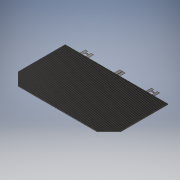
# Autodesk Inventor part: Part1
Saved by Autodesk Inventor 2017 (Build 210142000, 142)
## iProperties
Created: 2018-02-04
Part Number: Part1
Material: Glass
Document SubType Name: Modeling
Designer: Bradley
Density: 2.18 g/cm^3
Appearance: Semi-Polished
Author: Bradley
Autodesk Inventor part; units mm, degrees
ref_plane "YZ Plane" through (0, 0, 0) normal (1, 0, 0) x (0, 1, 0)
ref_plane "XZ Plane" through (0, 0, 0) normal (0, 1, 0) x (-1, 0, 0)
ref_plane "XY Plane" through (0, 0, 0) normal (0, 0, 1) x (1, 0, 0)
sketch "Sketch1" plane through (0, 0, 0) normal (0, 0, 1) x (1, 0, 0)
  line L0 (-26.5, -19.825) -> (26.5, -19.825)
  line L1 (34.5, -11.825) -> (34.5, 19.825)
  line L2 (34.5, 19.825) -> (-34.5, 19.825)
  line L3 (-34.5, 19.825) -> (-34.5, -11.825)
  line L4 (-34.5, -19.825) -> (34.5, 19.825) construction
  line L5 (34.5, -19.825) -> (-34.5, 19.825) construction
  line L6 (-34.5, -11.825) -> (-26.5, -19.825)
  line L7 (34.5, -11.825) -> (26.5, -19.825)
  point P0 (0, 0)
  dimension "d0" = 69
  dimension "d1" = 39.65
  dimension "d2" = 8
  dimension "d3" = 8
  dimension "d4" = 8
  dimension "d5" = 8
  constraints: 16 end point, 4 point on line, 2 midpoint, 2 parallel, 1 horizontal, 1 perpendicular
  measures "d0" distance of L2.end L1.end
  measures "d1" distance of L2.end L4.start
  measures "d2" distance of L3.end L4.start
  measures "d3" distance of L0.start L4.start
  measures "d4" distance of L1.start L5.start
  measures "d5" distance of L0.end L5.start
extrude "Extrusion1" add sketch "Sketch1" along normal mid plane 0.4
sketch "Sketch2" plane through (0, 0, -0.2) normal (0, 0, -1) x (-1, 0, 0)
  line L0 (-34.5, 19.825) -> (-34.5, -11.825) projected
  line L1 (-34.5, -11.825) -> (-26.5, -19.825) projected
  line L2 (-26.5, -19.825) -> (26.5, -19.825) projected
  line L3 (26.5, -19.825) -> (34.5, -11.825) projected
  line L4 (34.5, -11.825) -> (34.5, 19.825) projected
  line L5 (34.5, 19.825) -> (-34.5, 19.825) projected
  line L6 (-34.5, 19.825) -> (34.5, 19.825) projected
  line L7 (-3.125, 19.825) -> (3.125, 19.825)
  line L8 (3.125, 19.825) -> (3.125, 13.575)
  line L9 (3.125, 13.575) -> (-3.125, 13.575)
  line L10 (-3.125, 13.575) -> (-3.125, 19.825)
  point P0 (0, 0)
  point P1 (0, 13.575)
  dimension "d8" = 6.25
  constraints: 8 end point, 2 parallel, 2 perpendicular, 1 horizontal, 1 midpoint, 1 point on line, 1 vertical alignment
  measures "d8" distance of L8.end L9.end
extrude "Extrusion2" add sketch "Sketch2" along normal blind 0.1 contours L5 L8 L9 L10
sketch "Sketch3" plane through (-34.5, 19.825, 0.2) normal (0, 1, 0) x (1, 0, 0)
  line L0 (0, 0) -> (0, 0.4) projected
  line L1 (69, 0) -> (0, 0) projected
  line L2 (69, 0.4) -> (69, 0) projected
  line L3 (37.625, 0.4) -> (69, 0.4) projected
  line L4 (37.625, 0.4) -> (37.625, 0.5) projected
  line L5 (31.375, 0.5) -> (37.625, 0.5) projected
  line L6 (31.375, 0.4) -> (31.375, 0.5) projected
  line L7 (0, 0.4) -> (31.375, 0.4) projected
  line L8 (53.875, 0.32) -> (59.475, 0.32)
  line L9 (59.475, 0.32) -> (59.475, 0.38)
  line L10 (59.475, 0.38) -> (53.875, 0.38)
  line L11 (53.875, 0.38) -> (53.875, 0.32)
  line L12 (9.525, 0.32) -> (15.125, 0.32)
  line L13 (15.125, 0.32) -> (15.125, 0.38)
  line L14 (15.125, 0.38) -> (9.525, 0.38)
  line L15 (9.525, 0.38) -> (9.525, 0.32)
  line L16 (8, 0) -> (61, 0) construction
  line L17 (34.5, 0) -> (34.5, 0.5) construction
  line L18 (32.625, 0.32) -> (36.375, 0.32)
  line L19 (36.375, 0.32) -> (36.375, 0.38)
  line L20 (36.375, 0.38) -> (32.625, 0.38)
  line L21 (32.625, 0.38) -> (32.625, 0.32)
  point P0 (34.5, 0.2)
  point P1 (34.5, 0.32)
  dimension "d11" = 5.6
  dimension "d12" = 0.06
  dimension "d13" = 38.75
  dimension "d14" = 0.02
  dimension "d15" = 3.75
  constraints: 26 end point, 6 parallel, 4 collinear, 3 horizontal, 3 midpoint, 3 perpendicular, 1 vertical alignment, 2 other
  measures "d11" distance of L10.end L9.end
  measures "d12" distance of L10.end L8.start
  measures "d13" distance between parallel lines of L13 L11
  measures "d14" distance between parallel lines of L3 L10
  measures "d15" distance of L19.end L20.end
extrude "Extrusion3" add sketch "Sketch3" along normal blind 10.5 contours L11 L10 L9 L8 | L15 L14 L13 L12 | L21 L20 L19 L18
sketch "Sketch4" plane through (-24.975, 19.825, -0.12) normal (0, 0, 1) x (1, 0, 0)
  line L0 (5.6, 0) -> (0, 0) projected
  line L1 (5.6, 0) -> (5.6, 10.5) projected
  line L2 (0, 10.5) -> (5.6, 10.5) projected
  line L3 (0, 0) -> (0, 10.5) projected
  line L4 (-9.525, 0) -> (21.85, 0) projected
  line L5 (1.6, 0) -> (4, 0)
  line L6 (4, 0) -> (4, 1.9)
  line L7 (4, 1.9) -> (1.6, 1.9)
  line L8 (1.6, 1.9) -> (1.6, 0)
  line L9 (1.6, 2.65) -> (4, 2.65)
  line L10 (4, 2.65) -> (4, 5.9)
  line L11 (4, 5.9) -> (1.6, 5.9)
  line L12 (1.6, 5.9) -> (1.6, 2.65)
  line L13 (0, 10.5) -> (5.6, 10.5) projected
  line L14 (1.6, 10.5) -> (4, 10.5)
  line L15 (4, 10.5) -> (4, 6.65)
  line L16 (4, 6.65) -> (1.6, 6.65)
  line L17 (1.6, 6.65) -> (1.6, 10.5)
  point P0 (24.975, -19.825)
  point P1 (2.8, 10.5)
  dimension "d18" = 1.6
  dimension "d19" = 0.75
  dimension "d20" = 0.75
  dimension "d21" = 3.25
  dimension "d22" = 1.9
  constraints: 24 end point, 6 parallel, 6 point on line, 3 horizontal, 3 perpendicular, 2 midpoint
  measures "d18" distance between parallel lines of L3 L17
  measures "d19" distance between parallel lines of L11 L16
  measures "d20" distance between parallel lines of L7 L9
  measures "d21" distance of L9.end L10.end
  measures "d22" distance of L5.end L6.end
extrude "Extrusion4" cut sketch "Sketch4" against normal through all contours L0 L8 L7 L6 | L15 L16 L17 L2 | L12 L11 L10 L9
sketch "Sketch5" plane through (-1.875, 19.825, -0.12) normal (0, 0, 1) x (1, 0, 0)
  line L0 (3.75, 0) -> (0, 0) projected
  line L1 (3.75, 0) -> (3.75, 10.5) projected
  line L2 (0, 10.5) -> (3.75, 10.5) projected
  line L3 (0, 0) -> (0, 10.5) projected
  line L4 (0, 10.5) -> (3.75, 10.5) projected
  line L5 (1.75, 10.5) -> (2, 10.5)
  line L6 (2, 10.5) -> (2, 7.25)
  line L7 (2, 7.25) -> (1.75, 7.25)
  line L8 (1.75, 7.25) -> (1.75, 10.5)
  line L9 (0, 0) -> (3.75, 0) projected
  line L10 (1.75, 0) -> (2, 0)
  line L11 (2, 0) -> (2, 6.25)
  line L12 (2, 6.25) -> (1.75, 6.25)
  line L13 (1.75, 6.25) -> (1.75, 0)
  point P0 (1.875, -19.825)
  point P1 (1.875, 10.5)
  point P2 (1.875, 10.5)
  dimension "d25" = 1.75
  dimension "d26" = 1
  dimension "d27" = 6.25
  constraints: 16 end point, 4 midpoint, 4 parallel, 4 point on line, 2 horizontal, 2 perpendicular
  measures "d25" distance between parallel lines of L3 L8
  measures "d26" distance between parallel lines of L12 L7
  measures "d27" distance of L10.end L11.end
extrude "Extrusion5" cut sketch "Sketch5" against normal through all contours L0 L13 L12 L11 | L6 L7 L8 L2
mirror "Mirror1" about plane through (0, 0, 0) normal (1, 0, 0) of "Extrusion4"
sketch "Sketch6" plane through (0, 0, 0.2) normal (0, 0, 1) x (1, 0, 0)
  line L0 (34.5, -11.825) -> (34.5, 19.825) projected
  line L1 (34.5, 19.825) -> (-34.5, 19.825) projected
  line L2 (-34.5, 19.825) -> (-34.5, -11.825) projected
  line L3 (-34.5, -11.825) -> (-26.5, -19.825) projected
  line L4 (-26.5, -19.825) -> (26.5, -19.825) projected
  line L5 (26.5, -19.825) -> (34.5, -11.825) projected
  line L6 (33.9, 19.325) -> (34.1, 19.325)
  line L7 (34.1, 19.325) -> (34.1, -19.625)
  line L8 (34.1, -19.625) -> (33.9, -19.625)
  line L9 (33.9, -19.625) -> (33.9, 19.325)
  point P0 (0, 0)
  dimension "d30" = 0.2
  dimension "d31" = 0.5
  dimension "d32" = 0.2
  dimension "d33" = 33.9
  constraints: 8 end point, 2 parallel, 1 horizontal, 1 perpendicular
  measures "d30" distance between parallel lines of L8 L4
  measures "d31" distance between parallel lines of L1 L6
  measures "d32" distance of L6.start L6.end
  measures "d33" distance from line of point (0, 0) L9
extrude "Extrusion6" add sketch "Sketch6" along normal blind 0.01 contours L7 L8 L9 L5 | L5 L9 L6 L7
pattern_linear "Rectangular Pattern1" count 69 spacing 1 along (-1, 0, 0) of "Extrusion6"
sketch "Sketch7" plane through (0, 0, 0.2) normal (0, 0, 1) x (1, 0, 0)
  line L0 (-33.9, 19.325) -> (-33.9, -12.425) projected
  line L1 (-33.9, -12.425) -> (-33.1, -13.225) projected
  line L2 (-33.1, -13.225) -> (-33.1, 19.325) projected
  line L3 (-33.1, 19.325) -> (-32.9, 19.325) projected
  line L4 (-32.9, 19.325) -> (-32.9, -13.425) projected
  line L5 (-32.9, -13.425) -> (-32.1, -14.225) projected
  line L6 (-32.1, -14.225) -> (-32.1, 19.325) projected
  line L7 (-32.1, 19.325) -> (-31.9, 19.325) projected
  line L8 (-31.9, 19.325) -> (-31.9, -14.425) projected
  line L9 (-31.9, -14.425) -> (-31.1, -15.225) projected
  line L10 (-31.1, -15.225) -> (-31.1, 19.325) projected
  line L11 (-31.1, 19.325) -> (-30.9, 19.325) projected
  line L12 (-30.9, 19.325) -> (-30.9, -15.425) projected
  line L13 (-30.9, -15.425) -> (-30.1, -16.225) projected
  line L14 (-30.1, -16.225) -> (-30.1, 19.325) projected
  line L15 (-30.1, 19.325) -> (-29.9, 19.325) projected
  line L16 (-29.9, 19.325) -> (-29.9, -16.425) projected
  line L17 (-29.9, -16.425) -> (-29.1, -17.225) projected
  line L18 (-29.1, -17.225) -> (-29.1, 19.325) projected
  line L19 (-29.1, 19.325) -> (-28.9, 19.325) projected
  line L20 (-28.9, 19.325) -> (-28.9, -17.425) projected
  line L21 (-28.9, -17.425) -> (-28.1, -18.225) projected
  line L22 (-28.1, -18.225) -> (-28.1, 19.325) projected
  line L23 (-28.1, 19.325) -> (-27.9, 19.325) projected
  line L24 (-27.9, 19.325) -> (-27.9, -18.425) projected
  line L25 (-27.9, -18.425) -> (-27.1, -19.225) projected
  line L26 (-27.1, -19.225) -> (-27.1, 19.325) projected
  line L27 (-27.1, 19.325) -> (-26.9, 19.325) projected
  line L28 (-26.9, 19.325) -> (-26.9, -19.425) projected
  line L29 (-26.9, -19.425) -> (-26.5, -19.825) projected
  line L30 (-26.5, -19.825) -> (26.5, -19.825) projected
  line L31 (26.5, -19.825) -> (26.9, -19.425) projected
  line L32 (26.9, -19.425) -> (26.9, 19.325) projected
  line L33 (26.9, 19.325) -> (27.1, 19.325) projected
  line L34 (27.1, 19.325) -> (27.1, -19.225) projected
  line L35 (27.1, -19.225) -> (27.9, -18.425) projected
  line L36 (27.9, -18.425) -> (27.9, 19.325) projected
  line L37 (27.9, 19.325) -> (28.1, 19.325) projected
  line L38 (28.1, 19.325) -> (28.1, -18.225) projected
  line L39 (28.1, -18.225) -> (28.9, -17.425) projected
  line L40 (28.9, -17.425) -> (28.9, 19.325) projected
  line L41 (28.9, 19.325) -> (29.1, 19.325) projected
  line L42 (29.1, 19.325) -> (29.1, -17.225) projected
  line L43 (29.1, -17.225) -> (29.9, -16.425) projected
  line L44 (29.9, -16.425) -> (29.9, 19.325) projected
  line L45 (29.9, 19.325) -> (30.1, 19.325) projected
  line L46 (30.1, 19.325) -> (30.1, -16.225) projected
  line L47 (30.1, -16.225) -> (30.9, -15.425) projected
  line L48 (30.9, -15.425) -> (30.9, 19.325) projected
  line L49 (30.9, 19.325) -> (31.1, 19.325) projected
  line L50 (31.1, 19.325) -> (31.1, -15.225) projected
  line L51 (31.1, -15.225) -> (31.9, -14.425) projected
  line L52 (31.9, -14.425) -> (31.9, 19.325) projected
  line L53 (31.9, 19.325) -> (32.1, 19.325) projected
  line L54 (32.1, 19.325) -> (32.1, -14.225) projected
  line L55 (32.1, -14.225) -> (32.9, -13.425) projected
  line L56 (32.9, -13.425) -> (32.9, 19.325) projected
  line L57 (32.9, 19.325) -> (33.1, 19.325) projected
  line L58 (33.1, 19.325) -> (33.1, -13.225) projected
  line L59 (33.1, -13.225) -> (33.9, -12.425) projected
  line L60 (33.9, -12.425) -> (33.9, 19.325) projected
  line L61 (33.9, 19.325) -> (34.1, 19.325) projected
  line L62 (34.1, 19.325) -> (34.1, -12.225) projected
  line L63 (34.1, -12.225) -> (34.5, -11.825) projected
  line L64 (34.5, -11.825) -> (34.5, 19.825) projected
  line L65 (34.5, 19.825) -> (-34.5, 19.825) projected
  line L66 (-34.5, 19.825) -> (-34.5, -11.825) projected
  line L67 (-34.5, -11.825) -> (-34.1, -12.225) projected
  line L68 (-34.1, -12.225) -> (-34.1, 19.325) projected
  line L69 (-34.1, 19.325) -> (-33.9, 19.325) projected
  line L70 (-25.9, 19.325) -> (-25.9, -19.625) projected
  line L71 (-25.9, -19.625) -> (-26.1, -19.625) projected
  line L72 (-26.1, -19.625) -> (-26.1, 19.325) projected
  line L73 (-26.1, 19.325) -> (-25.9, 19.325) projected
  line L74 (-24.9, 19.325) -> (-24.9, -19.625) projected
  line L75 (-24.9, -19.625) -> (-25.1, -19.625) projected
  line L76 (-25.1, -19.625) -> (-25.1, 19.325) projected
  line L77 (-25.1, 19.325) -> (-24.9, 19.325) projected
  line L78 (-23.9, 19.325) -> (-23.9, -19.625) projected
  line L79 (-23.9, -19.625) -> (-24.1, -19.625) projected
  line L80 (-24.1, -19.625) -> (-24.1, 19.325) projected
  line L81 (-24.1, 19.325) -> (-23.9, 19.325) projected
  line L82 (-22.9, 19.325) -> (-22.9, -19.625) projected
  line L83 (-22.9, -19.625) -> (-23.1, -19.625) projected
  line L84 (-23.1, -19.625) -> (-23.1, 19.325) projected
  line L85 (-23.1, 19.325) -> (-22.9, 19.325) projected
  line L86 (-21.9, 19.325) -> (-21.9, -19.625) projected
  line L87 (-21.9, -19.625) -> (-22.1, -19.625) projected
  line L88 (-22.1, -19.625) -> (-22.1, 19.325) projected
  line L89 (-22.1, 19.325) -> (-21.9, 19.325) projected
  line L90 (-20.9, 19.325) -> (-20.9, -19.625) projected
  line L91 (-20.9, -19.625) -> (-21.1, -19.625) projected
  line L92 (-21.1, -19.625) -> (-21.1, 19.325) projected
  line L93 (-21.1, 19.325) -> (-20.9, 19.325) projected
  line L94 (-19.9, 19.325) -> (-19.9, -19.625) projected
  line L95 (-19.9, -19.625) -> (-20.1, -19.625) projected
  line L96 (-20.1, -19.625) -> (-20.1, 19.325) projected
  line L97 (-20.1, 19.325) -> (-19.9, 19.325) projected
  line L98 (-18.9, 19.325) -> (-18.9, -19.625) projected
  line L99 (-18.9, -19.625) -> (-19.1, -19.625) projected
  line L100 (-19.1, -19.625) -> (-19.1, 19.325) projected
  line L101 (-19.1, 19.325) -> (-18.9, 19.325) projected
  line L102 (-17.9, 19.325) -> (-17.9, -19.625) projected
  line L103 (-17.9, -19.625) -> (-18.1, -19.625) projected
  line L104 (-18.1, -19.625) -> (-18.1, 19.325) projected
  line L105 (-18.1, 19.325) -> (-17.9, 19.325) projected
  line L106 (-16.9, 19.325) -> (-16.9, -19.625) projected
  line L107 (-16.9, -19.625) -> (-17.1, -19.625) projected
  line L108 (-17.1, -19.625) -> (-17.1, 19.325) projected
  line L109 (-17.1, 19.325) -> (-16.9, 19.325) projected
  line L110 (-15.9, 19.325) -> (-15.9, -19.625) projected
  line L111 (-15.9, -19.625) -> (-16.1, -19.625) projected
  line L112 (-16.1, -19.625) -> (-16.1, 19.325) projected
  line L113 (-16.1, 19.325) -> (-15.9, 19.325) projected
  line L114 (-14.9, 19.325) -> (-14.9, -19.625) projected
  line L115 (-14.9, -19.625) -> (-15.1, -19.625) projected
  line L116 (-15.1, -19.625) -> (-15.1, 19.325) projected
  line L117 (-15.1, 19.325) -> (-14.9, 19.325) projected
  line L118 (-13.9, 19.325) -> (-13.9, -19.625) projected
  line L119 (-13.9, -19.625) -> (-14.1, -19.625) projected
  line L120 (-14.1, -19.625) -> (-14.1, 19.325) projected
  line L121 (-14.1, 19.325) -> (-13.9, 19.325) projected
  line L122 (-12.9, 19.325) -> (-12.9, -19.625) projected
  line L123 (-12.9, -19.625) -> (-13.1, -19.625) projected
  line L124 (-13.1, -19.625) -> (-13.1, 19.325) projected
  line L125 (-13.1, 19.325) -> (-12.9, 19.325) projected
  line L126 (-11.9, 19.325) -> (-11.9, -19.625) projected
  line L127 (-11.9, -19.625) -> (-12.1, -19.625) projected
  line L128 (-12.1, -19.625) -> (-12.1, 19.325) projected
  line L129 (-12.1, 19.325) -> (-11.9, 19.325) projected
  line L130 (-10.9, 19.325) -> (-10.9, -19.625) projected
  line L131 (-10.9, -19.625) -> (-11.1, -19.625) projected
  line L132 (-11.1, -19.625) -> (-11.1, 19.325) projected
  line L133 (-11.1, 19.325) -> (-10.9, 19.325) projected
  line L134 (-9.9, 19.325) -> (-9.9, -19.625) projected
  line L135 (-9.9, -19.625) -> (-10.1, -19.625) projected
  line L136 (-10.1, -19.625) -> (-10.1, 19.325) projected
  line L137 (-10.1, 19.325) -> (-9.9, 19.325) projected
  line L138 (-8.9, 19.325) -> (-8.9, -19.625) projected
  line L139 (-8.9, -19.625) -> (-9.1, -19.625) projected
  line L140 (-9.1, -19.625) -> (-9.1, 19.325) projected
  line L141 (-9.1, 19.325) -> (-8.9, 19.325) projected
  line L142 (-7.9, 19.325) -> (-7.9, -19.625) projected
  line L143 (-7.9, -19.625) -> (-8.1, -19.625) projected
  line L144 (-8.1, -19.625) -> (-8.1, 19.325) projected
  line L145 (-8.1, 19.325) -> (-7.9, 19.325) projected
  line L146 (-6.9, 19.325) -> (-6.9, -19.625) projected
  line L147 (-6.9, -19.625) -> (-7.1, -19.625) projected
  line L148 (-7.1, -19.625) -> (-7.1, 19.325) projected
  line L149 (-7.1, 19.325) -> (-6.9, 19.325) projected
  line L150 (-5.9, 19.325) -> (-5.9, -19.625) projected
  line L151 (-5.9, -19.625) -> (-6.1, -19.625) projected
  line L152 (-6.1, -19.625) -> (-6.1, 19.325) projected
  line L153 (-6.1, 19.325) -> (-5.9, 19.325) projected
  line L154 (-4.9, 19.325) -> (-4.9, -19.625) projected
  line L155 (-4.9, -19.625) -> (-5.1, -19.625) projected
  line L156 (-5.1, -19.625) -> (-5.1, 19.325) projected
  line L157 (-5.1, 19.325) -> (-4.9, 19.325) projected
  line L158 (-3.9, 19.325) -> (-3.9, -19.625) projected
  line L159 (-3.9, -19.625) -> (-4.1, -19.625) projected
  line L160 (-4.1, -19.625) -> (-4.1, 19.325) projected
  line L161 (-4.1, 19.325) -> (-3.9, 19.325) projected
  line L162 (-2.9, 19.325) -> (-2.9, -19.625) projected
  line L163 (-2.9, -19.625) -> (-3.1, -19.625) projected
  line L164 (-3.1, -19.625) -> (-3.1, 19.325) projected
  line L165 (-3.1, 19.325) -> (-2.9, 19.325) projected
  line L166 (-1.9, 19.325) -> (-1.9, -19.625) projected
  line L167 (-1.9, -19.625) -> (-2.1, -19.625) projected
  line L168 (-2.1, -19.625) -> (-2.1, 19.325) projected
  line L169 (-2.1, 19.325) -> (-1.9, 19.325) projected
  line L170 (-0.9, 19.325) -> (-0.9, -19.625) projected
  line L171 (-0.9, -19.625) -> (-1.1, -19.625) projected
  line L172 (-1.1, -19.625) -> (-1.1, 19.325) projected
  line L173 (-1.1, 19.325) -> (-0.9, 19.325) projected
  line L174 (0.1, 19.325) -> (0.1, -19.625) projected
  line L175 (0.1, -19.625) -> (-0.1, -19.625) projected
  line L176 (-0.1, -19.625) -> (-0.1, 19.325) projected
  line L177 (-0.1, 19.325) -> (0.1, 19.325) projected
  line L178 (1.1, 19.325) -> (1.1, -19.625) projected
  line L179 (1.1, -19.625) -> (0.9, -19.625) projected
  line L180 (0.9, -19.625) -> (0.9, 19.325) projected
  line L181 (0.9, 19.325) -> (1.1, 19.325) projected
  line L182 (2.1, 19.325) -> (2.1, -19.625) projected
  line L183 (2.1, -19.625) -> (1.9, -19.625) projected
  line L184 (1.9, -19.625) -> (1.9, 19.325) projected
  line L185 (1.9, 19.325) -> (2.1, 19.325) projected
  line L186 (3.1, 19.325) -> (3.1, -19.625) projected
  line L187 (3.1, -19.625) -> (2.9, -19.625) projected
  line L188 (2.9, -19.625) -> (2.9, 19.325) projected
  line L189 (2.9, 19.325) -> (3.1, 19.325) projected
  line L190 (4.1, 19.325) -> (4.1, -19.625) projected
  line L191 (4.1, -19.625) -> (3.9, -19.625) projected
  line L192 (3.9, -19.625) -> (3.9, 19.325) projected
  line L193 (3.9, 19.325) -> (4.1, 19.325) projected
  line L194 (5.1, 19.325) -> (5.1, -19.625) projected
  line L195 (5.1, -19.625) -> (4.9, -19.625) projected
  line L196 (4.9, -19.625) -> (4.9, 19.325) projected
  line L197 (4.9, 19.325) -> (5.1, 19.325) projected
  line L198 (6.1, 19.325) -> (6.1, -19.625) projected
  line L199 (6.1, -19.625) -> (5.9, -19.625) projected
  line L200 (5.9, -19.625) -> (5.9, 19.325) projected
  line L201 (5.9, 19.325) -> (6.1, 19.325) projected
  line L202 (7.1, 19.325) -> (7.1, -19.625) projected
  line L203 (7.1, -19.625) -> (6.9, -19.625) projected
  line L204 (6.9, -19.625) -> (6.9, 19.325) projected
  line L205 (6.9, 19.325) -> (7.1, 19.325) projected
  line L206 (8.1, 19.325) -> (8.1, -19.625) projected
  line L207 (8.1, -19.625) -> (7.9, -19.625) projected
  line L208 (7.9, -19.625) -> (7.9, 19.325) projected
  line L209 (7.9, 19.325) -> (8.1, 19.325) projected
  line L210 (9.1, 19.325) -> (9.1, -19.625) projected
  line L211 (9.1, -19.625) -> (8.9, -19.625) projected
  line L212 (8.9, -19.625) -> (8.9, 19.325) projected
  line L213 (8.9, 19.325) -> (9.1, 19.325) projected
  line L214 (10.1, 19.325) -> (10.1, -19.625) projected
  line L215 (10.1, -19.625) -> (9.9, -19.625) projected
  line L216 (9.9, -19.625) -> (9.9, 19.325) projected
  line L217 (9.9, 19.325) -> (10.1, 19.325) projected
  line L218 (11.1, 19.325) -> (11.1, -19.625) projected
  line L219 (11.1, -19.625) -> (10.9, -19.625) projected
  line L220 (10.9, -19.625) -> (10.9, 19.325) projected
  line L221 (10.9, 19.325) -> (11.1, 19.325) projected
  line L222 (12.1, 19.325) -> (12.1, -19.625) projected
  line L223 (12.1, -19.625) -> (11.9, -19.625) projected
  line L224 (11.9, -19.625) -> (11.9, 19.325) projected
  line L225 (11.9, 19.325) -> (12.1, 19.325) projected
  line L226 (13.1, 19.325) -> (13.1, -19.625) projected
  line L227 (13.1, -19.625) -> (12.9, -19.625) projected
  line L228 (12.9, -19.625) -> (12.9, 19.325) projected
  line L229 (12.9, 19.325) -> (13.1, 19.325) projected
  line L230 (14.1, 19.325) -> (14.1, -19.625) projected
  line L231 (14.1, -19.625) -> (13.9, -19.625) projected
  line L232 (13.9, -19.625) -> (13.9, 19.325) projected
  line L233 (13.9, 19.325) -> (14.1, 19.325) projected
  line L234 (15.1, 19.325) -> (15.1, -19.625) projected
  line L235 (15.1, -19.625) -> (14.9, -19.625) projected
  line L236 (14.9, -19.625) -> (14.9, 19.325) projected
  line L237 (14.9, 19.325) -> (15.1, 19.325) projected
  line L238 (16.1, 19.325) -> (16.1, -19.625) projected
  line L239 (16.1, -19.625) -> (15.9, -19.625) projected
  line L240 (15.9, -19.625) -> (15.9, 19.325) projected
  line L241 (15.9, 19.325) -> (16.1, 19.325) projected
  line L242 (17.1, 19.325) -> (17.1, -19.625) projected
  line L243 (17.1, -19.625) -> (16.9, -19.625) projected
  line L244 (16.9, -19.625) -> (16.9, 19.325) projected
  line L245 (16.9, 19.325) -> (17.1, 19.325) projected
  line L246 (18.1, 19.325) -> (18.1, -19.625) projected
  line L247 (18.1, -19.625) -> (17.9, -19.625) projected
  line L248 (17.9, -19.625) -> (17.9, 19.325) projected
  line L249 (17.9, 19.325) -> (18.1, 19.325) projected
  line L250 (19.1, 19.325) -> (19.1, -19.625) projected
  line L251 (19.1, -19.625) -> (18.9, -19.625) projected
  line L252 (18.9, -19.625) -> (18.9, 19.325) projected
  line L253 (18.9, 19.325) -> (19.1, 19.325) projected
  line L254 (20.1, 19.325) -> (20.1, -19.625) projected
  line L255 (20.1, -19.625) -> (19.9, -19.625) projected
  line L256 (19.9, -19.625) -> (19.9, 19.325) projected
  line L257 (19.9, 19.325) -> (20.1, 19.325) projected
  line L258 (21.1, 19.325) -> (21.1, -19.625) projected
  line L259 (21.1, -19.625) -> (20.9, -19.625) projected
  line L260 (20.9, -19.625) -> (20.9, 19.325) projected
  line L261 (20.9, 19.325) -> (21.1, 19.325) projected
  line L262 (22.1, 19.325) -> (22.1, -19.625) projected
  line L263 (22.1, -19.625) -> (21.9, -19.625) projected
  line L264 (21.9, -19.625) -> (21.9, 19.325) projected
  line L265 (21.9, 19.325) -> (22.1, 19.325) projected
  line L266 (23.1, 19.325) -> (23.1, -19.625) projected
  line L267 (23.1, -19.625) -> (22.9, -19.625) projected
  line L268 (22.9, -19.625) -> (22.9, 19.325) projected
  line L269 (22.9, 19.325) -> (23.1, 19.325) projected
  line L270 (24.1, 19.325) -> (24.1, -19.625) projected
  line L271 (24.1, -19.625) -> (23.9, -19.625) projected
  line L272 (23.9, -19.625) -> (23.9, 19.325) projected
  line L273 (23.9, 19.325) -> (24.1, 19.325) projected
  line L274 (25.1, 19.325) -> (25.1, -19.625) projected
  line L275 (25.1, -19.625) -> (24.9, -19.625) projected
  line L276 (24.9, -19.625) -> (24.9, 19.325) projected
  line L277 (24.9, 19.325) -> (25.1, 19.325) projected
  line L278 (26.1, 19.325) -> (26.1, -19.625) projected
  line L279 (26.1, -19.625) -> (25.9, -19.625) projected
  line L280 (25.9, -19.625) -> (25.9, 19.325) projected
  line L281 (25.9, 19.325) -> (26.1, 19.325) projected
  line L282 (-34.5, -11.5422) -> (-26.2172, -19.825)
  line L283 (34.5, -11.5422) -> (26.2172, -19.825)
  line L284 (-34.1, -12.225) -> (-33.9, -12.425) projected
  line L285 (-33.9, -12.425) -> (-33.9, -19.625) projected
  line L286 (-33.9, -19.625) -> (-34.1, -19.625) projected
  line L287 (-34.1, -19.625) -> (-34.1, -12.225) projected
  line L288 (-33.1, -13.225) -> (-32.9, -13.425) projected
  line L289 (-32.9, -13.425) -> (-32.9, -19.625) projected
  line L290 (-32.9, -19.625) -> (-33.1, -19.625) projected
  line L291 (-33.1, -19.625) -> (-33.1, -13.225) projected
  line L292 (-32.1, -14.225) -> (-31.9, -14.425) projected
  line L293 (-31.9, -14.425) -> (-31.9, -19.625) projected
  line L294 (-31.9, -19.625) -> (-32.1, -19.625) projected
  line L295 (-32.1, -19.625) -> (-32.1, -14.225) projected
  line L296 (-31.1, -15.225) -> (-30.9, -15.425) projected
  line L297 (-30.9, -15.425) -> (-30.9, -19.625) projected
  line L298 (-30.9, -19.625) -> (-31.1, -19.625) projected
  line L299 (-31.1, -19.625) -> (-31.1, -15.225) projected
  line L300 (-30.1, -16.225) -> (-29.9, -16.425) projected
  line L301 (-29.9, -16.425) -> (-29.9, -19.625) projected
  line L302 (-29.9, -19.625) -> (-30.1, -19.625) projected
  line L303 (-30.1, -19.625) -> (-30.1, -16.225) projected
  line L304 (-29.1, -17.225) -> (-28.9, -17.425) projected
  line L305 (-28.9, -17.425) -> (-28.9, -19.625) projected
  line L306 (-28.9, -19.625) -> (-29.1, -19.625) projected
  line L307 (-29.1, -19.625) -> (-29.1, -17.225) projected
  line L308 (-28.1, -18.225) -> (-27.9, -18.425) projected
  line L309 (-27.9, -18.425) -> (-27.9, -19.625) projected
  line L310 (-27.9, -19.625) -> (-28.1, -19.625) projected
  line L311 (-28.1, -19.625) -> (-28.1, -18.225) projected
  line L312 (-27.1, -19.225) -> (-26.9, -19.425) projected
  line L313 (-26.9, -19.425) -> (-26.9, -19.625) projected
  line L314 (-26.9, -19.625) -> (-27.1, -19.625) projected
  line L315 (-27.1, -19.625) -> (-27.1, -19.225) projected
  line L316 (33.9, -12.425) -> (34.1, -12.225) projected
  line L317 (34.1, -12.225) -> (34.1, -19.625) projected
  line L318 (34.1, -19.625) -> (33.9, -19.625) projected
  line L319 (33.9, -19.625) -> (33.9, -12.425) projected
  line L320 (32.9, -13.425) -> (33.1, -13.225) projected
  line L321 (33.1, -13.225) -> (33.1, -19.625) projected
  line L322 (33.1, -19.625) -> (32.9, -19.625) projected
  line L323 (32.9, -19.625) -> (32.9, -13.425) projected
  line L324 (31.9, -14.425) -> (32.1, -14.225) projected
  line L325 (32.1, -14.225) -> (32.1, -19.625) projected
  line L326 (32.1, -19.625) -> (31.9, -19.625) projected
  line L327 (31.9, -19.625) -> (31.9, -14.425) projected
  line L328 (30.9, -15.425) -> (31.1, -15.225) projected
  line L329 (31.1, -15.225) -> (31.1, -19.625) projected
  line L330 (31.1, -19.625) -> (30.9, -19.625) projected
  line L331 (30.9, -19.625) -> (30.9, -15.425) projected
  line L332 (29.9, -16.425) -> (30.1, -16.225) projected
  line L333 (30.1, -16.225) -> (30.1, -19.625) projected
  line L334 (30.1, -19.625) -> (29.9, -19.625) projected
  line L335 (29.9, -19.625) -> (29.9, -16.425) projected
  line L336 (28.9, -17.425) -> (29.1, -17.225) projected
  line L337 (29.1, -17.225) -> (29.1, -19.625) projected
  line L338 (29.1, -19.625) -> (28.9, -19.625) projected
  line L339 (28.9, -19.625) -> (28.9, -17.425) projected
  line L340 (27.9, -18.425) -> (28.1, -18.225) projected
  line L341 (28.1, -18.225) -> (28.1, -19.625) projected
  line L342 (28.1, -19.625) -> (27.9, -19.625) projected
  line L343 (27.9, -19.625) -> (27.9, -18.425) projected
  line L344 (26.9, -19.425) -> (27.1, -19.225) projected
  line L345 (27.1, -19.225) -> (27.1, -19.625) projected
  line L346 (27.1, -19.625) -> (26.9, -19.625) projected
  line L347 (26.9, -19.625) -> (26.9, -19.425) projected
  line L348 (-34.5, -11.825) -> (-26.5, -19.825)
  line L349 (34.5, -11.825) -> (26.5, -19.825)
  line L350 (-26.5, -19.825) -> (26.5, -19.825) projected
  line L351 (26.2172, -19.825) -> (26.5, -19.825)
  line L352 (34.5, 19.825) -> (34.5, -11.825) projected
  line L353 (34.5, -11.5422) -> (34.5, -11.825)
  line L354 (-26.5, -19.825) -> (-26.2172, -19.825)
  line L355 (-34.5, -11.5422) -> (-34.5, -11.825)
  point P0 (0, 0)
  dimension "d39" = 0.2
  dimension "d40" = 0.2
  constraints: 16 end point, 4 point on line, 2 parallel, 2 perpendicular, 1 collinear, 1 horizontal, 1 vertical
  measures "d39" distance between parallel lines of L29 L282
  measures "d40" distance between parallel lines of L31 L283
extrude "Extrusion7" cut sketch "Sketch7" along normal blind 0.01 contours L282 L2 L1 L0 | L0 L284 L68 L282 | L285 L286 L287 L284 | L68 L67 L66 L282 | L282 L4 L288 L2 | L288 L289 L290 L291 | L282 L6 L5 L4 | L282 L8 L292 L6 | L292 L293 L294 L295 | L282 L10 L9 L8 | L64 L63 L62 L283 | L282 L12 L296 L10 | L296 L297 L298 L299 | L62 L316 L60 L283 | L282 L14 L13 L12 | L317 L318 L319 L316 | L60 L59 L58 L283 | L282 L16 L300 L14 | L300 L301 L302 L303 | L58 L320 L56 L283 | L282 L18 L17 L16 | L321 L322 L323 L320 | L56 L55 L54 L283 | L282 L20 L304 L18 | L304 L305 L306 L307 | L54 L324 L52 L283 | L282 L22 L21 L20 | L325 L326 L327 L324 | L52 L51 L50 L283 | L282 L24 L308 L22 | L308 L309 L310 L311 | L50 L328 L48 L283 | L282 L26 L25 L24 | L329 L330 L331 L328 | L48 L47 L46 L283 | L282 L28 L312 L26 | L312 L313 L314 L315 | L46 L332 L44 L283 | L282 L30 L29 L28 | L333 L334 L335 L332 | L44 L43 L42 L283 | L42 L336 L40 L283 | L283 L32 L31 L30 | L337 L338 L339 L336 | L40 L39 L38 L283 | L283 L34 L344 L32 | L38 L340 L36 L283 | L344 L345 L346 L347 | L283 L36 L35 L34 | L341 L342 L343 L340
sketch "Sketch8" plane through (-19.375, 19.825, -0.12) normal (0, 0, 1) x (1, 0, 0)
  line L0 (-1.6, 5.9) -> (-1.6, 2.65) projected
  line L1 (-1.6, 2.65) -> (-4, 2.65) projected
  line L2 (-4, 2.65) -> (-4, 5.9) projected
  line L3 (-4, 5.9) -> (-1.6, 5.9) projected
  line L4 (-4, 0) -> (-4, 1.9) projected
  line L5 (-4, 1.9) -> (-1.6, 1.9) projected
  line L6 (-1.6, 1.9) -> (-1.6, 0) projected
  line L7 (0, 0) -> (-1.6, 0) projected
  line L8 (0, 0) -> (0, 10.5) projected
  line L9 (-1.6, 10.5) -> (0, 10.5) projected
  line L10 (-1.6, 10.5) -> (-1.6, 6.65) projected
  line L11 (-1.6, 6.65) -> (-4, 6.65) projected
  line L12 (-4, 6.65) -> (-4, 10.5) projected
  line L13 (-5.6, 10.5) -> (-4, 10.5) projected
  line L14 (-5.6, 0) -> (-5.6, 10.5) projected
  line L15 (-4, 0) -> (-5.6, 0) projected
  line L16 (19.25, 7.25) -> (19.25, 10.5) projected
  line L17 (17.5, 10.5) -> (19.25, 10.5) projected
  line L18 (17.5, 0) -> (17.5, 10.5) projected
  line L19 (19.25, 0) -> (17.5, 0) projected
  line L20 (19.25, 0) -> (19.25, 6.25) projected
  line L21 (19.25, 6.25) -> (19.5, 6.25) projected
  line L22 (19.5, 6.25) -> (19.5, 0) projected
  line L23 (21.25, 0) -> (19.5, 0) projected
  line L24 (21.25, 0) -> (21.25, 10.5) projected
  line L25 (19.5, 10.5) -> (21.25, 10.5) projected
  line L26 (19.5, 10.5) -> (19.5, 7.25) projected
  line L27 (19.5, 7.25) -> (19.25, 7.25) projected
  line L28 (40.35, 6.65) -> (40.35, 10.5) projected
  line L29 (38.75, 10.5) -> (40.35, 10.5) projected
  line L30 (38.75, 0) -> (38.75, 10.5) projected
  line L31 (40.35, 0) -> (38.75, 0) projected
  line L32 (40.35, 0) -> (40.35, 1.9) projected
  line L33 (40.35, 1.9) -> (42.75, 1.9) projected
  line L34 (42.75, 1.9) -> (42.75, 0) projected
  line L35 (44.35, 0) -> (42.75, 0) projected
  line L36 (44.35, 0) -> (44.35, 10.5) projected
  line L37 (42.75, 10.5) -> (44.35, 10.5) projected
  line L38 (42.75, 10.5) -> (42.75, 6.65) projected
  line L39 (42.75, 6.65) -> (40.35, 6.65) projected
  line L40 (42.75, 5.9) -> (42.75, 2.65) projected
  line L41 (42.75, 2.65) -> (40.35, 2.65) projected
  line L42 (40.35, 2.65) -> (40.35, 5.9) projected
  line L43 (40.35, 5.9) -> (42.75, 5.9) projected
  line L44 (-5.6, 10.5) -> (44.35, 10.5)
  line L45 (44.35, 10.5) -> (44.35, 4)
  line L46 (44.35, 4) -> (-5.6, 4)
  line L47 (-5.6, 4) -> (-5.6, 10.5)
  point P0 (19.375, -19.825)
  dimension "d43" = 4
  constraints: 8 end point, 2 parallel, 1 horizontal, 1 perpendicular, 1 point on line
  measures "d43" distance between parallel lines of L46 L35
extrude "Extrusion8" cut sketch "Sketch8" against normal through all contours L3 L2 L46 L14 L13 L12 L11 L10 L9 L8 L0 | L0 L46 L2 L3 | L8 L44 L18 L46 | L18 L17 L16 L27 L26 L25 L24 L46 L22 L21 L20 | L10 L11 L12 L44 | L20 L21 L22 L46 | L44 L26 L27 L16 | L24 L44 L30 L46 | L30 L29 L28 L39 L38 L37 L36 L46 L40 L43 L42 | L42 L43 L40 L46 | L44 L38 L39 L28
equation "\"d3\" = d2"
equation "\"d4\" = d2"
equation "\"d5\" = d4"
equation "\"d20\" = d19"
equation "\"d40\" = d39"
body "Solid1"
